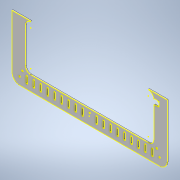
# Autodesk Inventor part: BackAcrylicPlate
Saved by Autodesk Inventor 2022 (Build 260153000, 153)
## iProperties
Created: 2021-04-22
Part Number: BackAcrylicPlate
Material: Generic
Document SubType Name: Modeling
Designer: Viktor
Density: 1 g/cm^3
Appearance: Default
Author: Viktor
Autodesk Inventor part; units mm, degrees
ref_plane "YZ Plane" through (0, 0, 0) normal (1, 0, 0) x (0, 1, 0)
ref_plane "XZ Plane" through (0, 0, 0) normal (0, 1, 0) x (-1, 0, 0)
ref_plane "XY Plane" through (0, 0, 0) normal (0, 0, 1) x (1, 0, 0)
sketch "Sketch1" plane through (0, 0, 0) normal (0, 0, 1) x (1, 0, 0)
  line L0 (-222.5, -24) -> (222.5, -24)
  line L1 (222.5, -24) -> (222.5, 24)
  line L2 (222.5, 24) -> (-222.5, 24)
  line L3 (-222.5, 24) -> (-222.5, -24)
  line L4 (-222.5, -24) -> (222.5, 24) construction
  line L5 (222.5, -24) -> (-222.5, 24) construction
  point P0 (0, 0)
  dimension "d0" = 445
  dimension "d1" = 48
  constraints: 12 end point, 2 midpoint, 2 parallel, 1 horizontal, 1 perpendicular
  measures "d0" distance of L1.end L2.end
  measures "d1" distance of L2.end L0.start
extrude "Extrusion1" add sketch "Sketch1" along normal blind 3
fillet "Fillet1" radius 22 2 edges at (-222.5, -24, 1.5) (222.5, -24, 1.5)
sketch "Sketch2" plane through (0, 0, 3) normal (0, 0, 1) x (1, 0, 0)
  line L0 (-311.5, 0) -> (311.5, 0) projected
  line L1 (0, -9) -> (0, 9) construction
  line L2 (-2, -9) -> (-2, 9)
  line L3 (2, 9) -> (2, -9)
  arc A0 (-2, -9) -> (2, -9) centre (0, -9) ccw
  arc A1 (2, 9) -> (-2, 9) centre (0, 9) ccw
  point P0 (0, 0)
  dimension "d5" = 18
  dimension "d6" = 2
  constraints: 8 end point, 4 point on circle, 4 tangent, 2 centre point, 1 midpoint, 1 parallel, 1 perpendicular
  measures "d5" distance of L3.start L3.end
  measures "d6" radius of A1
extrude "Extrusion2" cut sketch "Sketch2" against normal blind 3
pattern_linear "Rectangular Pattern1" count 10 spacing 20 along (-1, 0, 0) count 10 spacing 20 along (1, 0, 0) of "Extrusion2"
sketch "Sketch3" plane through (0, 0, 3) normal (0, 0, 1) x (1, 0, 0)
  arc A0 (-222.5, -2) -> (-200.5, -24) centre (-200.5, -2) ccw projected
  arc A1 (200.5, -24) -> (222.5, -2) centre (200.5, -2) ccw projected
  circle A2 centre (-200.5, -2) radius 2.25
  line L0 (0, 34.5113) -> (0, -39.0676) projected
  circle A3 centre (200.5, -2) radius 2.25
  point P0 (0, 0)
  dimension "d15" = 4.5
  constraints: 2 centre point, 1 coincident, 1 symmetric about line, 1 other
  measures "d15" diameter of A2
extrude "Extrusion3" cut sketch "Sketch3" against normal blind 3
fillet "Fillet2" radius 2 2 edges at (-222.5, 24, 1.5) (222.5, 24, 1.5)
sketch "Sketch7" plane through (0, 0, 3) normal (0, 0, 1) x (1, 0, 0)
  arc A0 (2, 9) -> (-2, 9) centre (0, 9) ccw projected
  line L0 (-2, -9) -> (-2, 9) projected
  arc A1 (-2, -9) -> (2, -9) centre (0, -9) ccw projected
  line L1 (2, 9) -> (2, -9) projected
  point P0 (0, 0)
extrude "Extrusion6" add sketch "Sketch7" against normal up to surface (3 mm away)
sketch "Sketch4" plane through (0, 0, 3) normal (0, 0, 1) x (1, 0, 0)
  circle A0 centre (-192.5, 16) radius 2.25
  line L0 (0, 33.6) -> (0, -33.6) projected
  line L1 (-222.5, 22) -> (-222.5, -2) projected
  line L2 (220.5, 24) -> (-220.5, 24) projected
  circle A1 centre (192.5, 16) radius 2.25
  circle A2 centre (0, 8) radius 2.25
  point P0 (0, 0)
  dimension "d19" = 4.5
  dimension "d20" = 30
  dimension "d21" = 8
  dimension "d24" = 4.5
  dimension "d25" = 16
  constraints: 3 centre point, 1 point on line, 1 symmetric about line, 1 other
  measures "d19" diameter of A0
  measures "d20" distance from line of L1 A0.centre
  measures "d21" distance from line of L2 A0.centre
  measures "d24" diameter of A2
  measures "d25" distance from line of L2 A2.centre
extrude "Extrusion4" cut sketch "Sketch4" against normal blind 3
sketch "Sketch6" plane through (0, 0, 3) normal (0, 0, 1) x (1, 0, 0)
  line L0 (0, -39.1505) -> (0, 35.0083) construction
  line L1 (-184, 40.8676) -> (184, 40.8676)
  line L2 (184, 40.8676) -> (184, 18)
  line L3 (184, 18) -> (-184, 18)
  line L4 (-184, 18) -> (-184, 40.8676)
  line L5 (-184, 40.8676) -> (184, 18) construction
  line L6 (184, 40.8676) -> (-184, 18) construction
  line L7 (220.5, 24) -> (-220.5, 24) projected
  point P0 (0, 0)
  point P1 (0, 29.4338)
  dimension "d26" = 6
  dimension "d27" = 368
  constraints: 12 end point, 2 midpoint, 2 parallel, 1 horizontal, 1 perpendicular, 1 point on line
  measures "d26" distance between parallel lines of L7 L3
  measures "d27" distance between parallel lines of L2 L4
extrude "Extrusion5" cut sketch "Sketch6" against normal through all
fillet "Fillet3" radius 1 2 edges at (-184, 18, 1.5) (184, 18, 1.5)
sketch "Sketch8" plane through (0, 0, 3) normal (0, 0, 1) x (1, 0, 0)
  line L0 (-222.5, 22) -> (-222.5, -2) projected
  line L1 (-222.5, 22) -> (-184, 22)
  line L2 (-184, 22) -> (-184, 151)
  line L3 (-184, 151) -> (-222.5, 151)
  line L4 (-222.5, 151) -> (-222.5, 22)
  line L5 (-184, 19) -> (-184, 24) projected
  line L6 (0, -64.6889) -> (0, 188.2392) projected
  line L7 (222.5, 22) -> (184, 22)
  line L8 (184, 22) -> (184, 151)
  line L9 (184, 151) -> (222.5, 151)
  line L10 (222.5, 151) -> (222.5, 22)
  line L11 (184, 19) -> (184, 24)
  line L12 (-184, 151) -> (-169, 151)
  line L13 (-169, 151) -> (-169, 149)
  line L14 (-169, 149) -> (-184, 149)
  line L15 (-184, 149) -> (-184, 151)
  line L16 (184, 151) -> (169, 151)
  line L17 (169, 151) -> (169, 149)
  line L18 (169, 149) -> (184, 149)
  point P0 (0, 0)
  point P1 (-184, 21.5)
  point P2 (184, 21.5)
  dimension "d33" = 129
  dimension "d34" = 15
  dimension "d35" = 2
  constraints: 32 end point, 10 symmetric about line, 4 parallel, 2 horizontal, 2 perpendicular, 2 point on line, 1 midpoint
  measures "d33" distance between parallel lines of L1 L3
  measures "d34" distance between parallel lines of L2 L13
  measures "d35" distance between parallel lines of L12 L14
extrude "Extrusion7" add sketch "Sketch8" against normal up to surface (3 mm away)
fillet "Fillet4" radius 15 2 edges at (-184, 149, 1.5) (184, 149, 1.5)
sketch "Sketch10" plane through (0, 0, 3) normal (0, 0, 1) x (1, 0, 0)
  line L0 (184, 136) -> (199, 136)
  line L1 (199, 136) -> (199, 121)
  line L2 (199, 121) -> (184, 121)
  line L3 (184, 121) -> (184, 136)
  line L4 (222.5, 151) -> (169, 151) projected
  point P0 (0, 0)
  dimension "d39" = 15
  dimension "d40" = 15
  dimension "d41" = 15
  constraints: 8 end point, 2 parallel, 1 horizontal, 1 perpendicular
  measures "d39" distance between parallel lines of L4 L0
  measures "d40" distance between parallel lines of L2 L0
  measures "d41" distance between parallel lines of L3 L1
extrude "Extrusion8" cut sketch "Sketch10" against normal blind 10
fillet "Fillet5" radius 2 3 edges at (184, 121, 1.5) (199, 121, 1.5) (199, 136, 1.5)
sketch "Sketch12" plane through (0, 0, 3) normal (0, 0, 1) x (1, 0, 0)
  circle A0 centre (-169, 33) radius 15
  line L0 (-184, 134) -> (-184, 19) projected
  arc A1 (186, 121) -> (184, 119) centre (186, 119) ccw projected
  line L1 (184, 119) -> (184, 19) projected
  arc A2 (183, 18) -> (184, 19) centre (183, 19) ccw projected
  line L2 (183, 18) -> (-183, 18) projected
  arc A3 (-184, 19) -> (-183, 18) centre (-183, 19) ccw projected
  line L3 (-184, 19) -> (-184, 134) projected
  arc A4 (-169, 149) -> (-184, 134) centre (-169, 134) ccw projected
  line L4 (-169, 149) -> (-169, 151) projected
  line L5 (-169, 151) -> (-222.5, 151) projected
  line L6 (-222.5, 151) -> (-222.5, -2) projected
  arc A5 (-222.5, -2) -> (-200.5, -24) centre (-200.5, -2) ccw projected
  line L7 (-200.5, -24) -> (200.5, -24) projected
  arc A6 (200.5, -24) -> (222.5, -2) centre (200.5, -2) ccw projected
  line L8 (222.5, -2) -> (222.5, 151) projected
  line L9 (222.5, 151) -> (169, 151) projected
  line L10 (169, 151) -> (169, 149) projected
  arc A7 (184, 134) -> (169, 149) centre (169, 134) ccw projected
  line L11 (184, 136) -> (197, 136) projected
  arc A8 (199, 134) -> (197, 136) centre (197, 134) ccw projected
  line L12 (199, 134) -> (199, 123) projected
  arc A9 (197, 121) -> (199, 123) centre (197, 123) ccw projected
  line L13 (197, 121) -> (186, 121) projected
  arc A10 (38, -9) -> (42, -9) centre (40, -9) ccw projected
  line L14 (38, -9) -> (38, 9) projected
  arc A11 (42, 9) -> (38, 9) centre (40, 9) ccw projected
  line L15 (42, 9) -> (42, -9) projected
  arc A12 (78, -9) -> (82, -9) centre (80, -9) ccw projected
  line L16 (78, -9) -> (78, 9) projected
  arc A13 (82, 9) -> (78, 9) centre (80, 9) ccw projected
  line L17 (82, 9) -> (82, -9) projected
  arc A14 (118, -9) -> (122, -9) centre (120, -9) ccw projected
  line L18 (118, -9) -> (118, 9) projected
  arc A15 (122, 9) -> (118, 9) centre (120, 9) ccw projected
  line L19 (122, 9) -> (122, -9) projected
  arc A16 (158, -9) -> (162, -9) centre (160, -9) ccw projected
  line L20 (158, -9) -> (158, 9) projected
  arc A17 (162, 9) -> (158, 9) centre (160, 9) ccw projected
  line L21 (162, 9) -> (162, -9) projected
  arc A18 (-22, -9) -> (-18, -9) centre (-20, -9) ccw projected
  line L22 (-22, -9) -> (-22, 9) projected
  arc A19 (-18, 9) -> (-22, 9) centre (-20, 9) ccw projected
  line L23 (-18, 9) -> (-18, -9) projected
  arc A20 (-42, -9) -> (-38, -9) centre (-40, -9) ccw projected
  line L24 (-42, -9) -> (-42, 9) projected
  arc A21 (-38, 9) -> (-42, 9) centre (-40, 9) ccw projected
  line L25 (-38, 9) -> (-38, -9) projected
  arc A22 (-62, -9) -> (-58, -9) centre (-60, -9) ccw projected
  line L26 (-62, -9) -> (-62, 9) projected
  arc A23 (-58, 9) -> (-62, 9) centre (-60, 9) ccw projected
  line L27 (-58, 9) -> (-58, -9) projected
  arc A24 (-82, -9) -> (-78, -9) centre (-80, -9) ccw projected
  line L28 (-82, -9) -> (-82, 9) projected
  arc A25 (-78, 9) -> (-82, 9) centre (-80, 9) ccw projected
  line L29 (-78, 9) -> (-78, -9) projected
  arc A26 (-102, -9) -> (-98, -9) centre (-100, -9) ccw projected
  line L30 (-102, -9) -> (-102, 9) projected
  arc A27 (-98, 9) -> (-102, 9) centre (-100, 9) ccw projected
  line L31 (-98, 9) -> (-98, -9) projected
  arc A28 (-122, -9) -> (-118, -9) centre (-120, -9) ccw projected
  line L32 (-122, -9) -> (-122, 9) projected
  arc A29 (-118, 9) -> (-122, 9) centre (-120, 9) ccw projected
  line L33 (-118, 9) -> (-118, -9) projected
  arc A30 (-142, -9) -> (-138, -9) centre (-140, -9) ccw projected
  line L34 (-142, -9) -> (-142, 9) projected
  arc A31 (-138, 9) -> (-142, 9) centre (-140, 9) ccw projected
  line L35 (-138, 9) -> (-138, -9) projected
  arc A32 (-162, -9) -> (-158, -9) centre (-160, -9) ccw projected
  line L36 (-162, -9) -> (-162, 9) projected
  arc A33 (-158, 9) -> (-162, 9) centre (-160, 9) ccw projected
  line L37 (-158, 9) -> (-158, -9) projected
  arc A34 (-182, -9) -> (-178, -9) centre (-180, -9) ccw projected
  line L38 (-182, -9) -> (-182, 9) projected
  arc A35 (-178, 9) -> (-182, 9) centre (-180, 9) ccw projected
  line L39 (-178, 9) -> (-178, -9) projected
  arc A36 (178, -9) -> (182, -9) centre (180, -9) ccw projected
  line L40 (178, -9) -> (178, 9) projected
  arc A37 (182, 9) -> (178, 9) centre (180, 9) ccw projected
  line L41 (182, 9) -> (182, -9) projected
  arc A38 (138, -9) -> (142, -9) centre (140, -9) ccw projected
  line L42 (138, -9) -> (138, 9) projected
  arc A39 (142, 9) -> (138, 9) centre (140, 9) ccw projected
  line L43 (142, 9) -> (142, -9) projected
  arc A40 (98, -9) -> (102, -9) centre (100, -9) ccw projected
  line L44 (98, -9) -> (98, 9) projected
  arc A41 (102, 9) -> (98, 9) centre (100, 9) ccw projected
  line L45 (102, 9) -> (102, -9) projected
  arc A42 (58, -9) -> (62, -9) centre (60, -9) ccw projected
  line L46 (58, -9) -> (58, 9) projected
  arc A43 (62, 9) -> (58, 9) centre (60, 9) ccw projected
  line L47 (62, 9) -> (62, -9) projected
  arc A44 (18, -9) -> (22, -9) centre (20, -9) ccw projected
  line L48 (18, -9) -> (18, 9) projected
  arc A45 (22, 9) -> (18, 9) centre (20, 9) ccw projected
  line L49 (22, 9) -> (22, -9) projected
  circle A46 centre (-200.5, -2) radius 2.25 projected
  circle A47 centre (200.5, -2) radius 2.25 projected
  circle A48 centre (0, 8) radius 2.25 projected
  circle A49 centre (-192.5, 16) radius 2.25 projected
  circle A50 centre (192.5, 16) radius 2.25 projected
  line L50 (183, 18) -> (-183, 18) projected
  line L51 (0, -64.6889) -> (0, 188.2392) projected
  circle A51 centre (169, 33) radius 15
  line L52 (184, 134) -> (184, 19)
  line L53 (-183, 18) -> (183, 18)
  arc A52 (183, 18) -> (184, 19) centre (183, 19) ccw
  line L54 (184, 19) -> (184, 134)
  arc A53 (142, 9) -> (138, 9) centre (140, 9) ccw
  arc A54 (162, 9) -> (158, 9) centre (160, 9) ccw
  arc A55 (182, 9) -> (178, 9) centre (180, 9) ccw
  line L55 (-183, 18) -> (183, 18)
  line L56 (184, 134) -> (184, 136) projected
  point P0 (0, 0)
  point P1 (184, 33)
  point P2 (169, 18)
  point P3 (-169, 18)
  point P4 (-184, 33)
  dimension "d45" = 30
  constraints: 11 symmetric about line, 8 end point, 8 point on circle, 6 centre point, 2 tangent, 5 other
  measures "d45" diameter of A0
extrude "Extrusion9" add sketch "Sketch12" against normal up to surface (3 mm away) contours A0 L2 A3 L0 | A51 L1 A2 L2
sketch "Sketch14" plane through (0, 0, 3) normal (0, 0, 1) x (1, 0, 0)
  arc A0 (186, 121) -> (184, 119) centre (186, 119) ccw projected
  line L0 (184, 119) -> (184, 33) projected
  arc A1 (169, 18) -> (184, 33) centre (169, 33) ccw projected
  line L1 (169, 18) -> (-169, 18) projected
  arc A2 (-184, 33) -> (-169, 18) centre (-169, 33) ccw projected
  line L2 (-184, 33) -> (-184, 134) projected
  arc A3 (-169, 149) -> (-184, 134) centre (-169, 134) ccw projected
  line L3 (-169, 149) -> (-169, 151) projected
  line L4 (-169, 151) -> (-222.5, 151) projected
  line L5 (-222.5, 151) -> (-222.5, -2) projected
  arc A4 (-222.5, -2) -> (-200.5, -24) centre (-200.5, -2) ccw projected
  line L6 (-200.5, -24) -> (200.5, -24) projected
  arc A5 (200.5, -24) -> (222.5, -2) centre (200.5, -2) ccw projected
  line L7 (222.5, -2) -> (222.5, 151) projected
  line L8 (222.5, 151) -> (169, 151) projected
  line L9 (169, 151) -> (169, 149) projected
  arc A6 (184, 134) -> (169, 149) centre (169, 134) ccw projected
  line L10 (184, 136) -> (197, 136) projected
  arc A7 (199, 134) -> (197, 136) centre (197, 134) ccw projected
  line L11 (199, 134) -> (199, 123) projected
  arc A8 (197, 121) -> (199, 123) centre (197, 123) ccw projected
  line L12 (197, 121) -> (186, 121) projected
  arc A9 (38, -9) -> (42, -9) centre (40, -9) ccw projected
  line L13 (38, -9) -> (38, 9) projected
  arc A10 (42, 9) -> (38, 9) centre (40, 9) ccw projected
  line L14 (42, 9) -> (42, -9) projected
  arc A11 (78, -9) -> (82, -9) centre (80, -9) ccw projected
  line L15 (78, -9) -> (78, 9) projected
  arc A12 (82, 9) -> (78, 9) centre (80, 9) ccw projected
  line L16 (82, 9) -> (82, -9) projected
  arc A13 (118, -9) -> (122, -9) centre (120, -9) ccw projected
  line L17 (118, -9) -> (118, 9) projected
  arc A14 (122, 9) -> (118, 9) centre (120, 9) ccw projected
  line L18 (122, 9) -> (122, -9) projected
  arc A15 (158, -9) -> (162, -9) centre (160, -9) ccw projected
  line L19 (158, -9) -> (158, 9) projected
  arc A16 (162, 9) -> (158, 9) centre (160, 9) ccw projected
  line L20 (162, 9) -> (162, -9) projected
  arc A17 (-22, -9) -> (-18, -9) centre (-20, -9) ccw projected
  line L21 (-22, -9) -> (-22, 9) projected
  arc A18 (-18, 9) -> (-22, 9) centre (-20, 9) ccw projected
  line L22 (-18, 9) -> (-18, -9) projected
  arc A19 (-42, -9) -> (-38, -9) centre (-40, -9) ccw projected
  line L23 (-42, -9) -> (-42, 9) projected
  arc A20 (-38, 9) -> (-42, 9) centre (-40, 9) ccw projected
  line L24 (-38, 9) -> (-38, -9) projected
  arc A21 (-62, -9) -> (-58, -9) centre (-60, -9) ccw projected
  line L25 (-62, -9) -> (-62, 9) projected
  arc A22 (-58, 9) -> (-62, 9) centre (-60, 9) ccw projected
  line L26 (-58, 9) -> (-58, -9) projected
  arc A23 (-82, -9) -> (-78, -9) centre (-80, -9) ccw projected
  line L27 (-82, -9) -> (-82, 9) projected
  arc A24 (-78, 9) -> (-82, 9) centre (-80, 9) ccw projected
  line L28 (-78, 9) -> (-78, -9) projected
  arc A25 (-102, -9) -> (-98, -9) centre (-100, -9) ccw projected
  line L29 (-102, -9) -> (-102, 9) projected
  arc A26 (-98, 9) -> (-102, 9) centre (-100, 9) ccw projected
  line L30 (-98, 9) -> (-98, -9) projected
  arc A27 (-122, -9) -> (-118, -9) centre (-120, -9) ccw projected
  line L31 (-122, -9) -> (-122, 9) projected
  arc A28 (-118, 9) -> (-122, 9) centre (-120, 9) ccw projected
  line L32 (-118, 9) -> (-118, -9) projected
  arc A29 (-142, -9) -> (-138, -9) centre (-140, -9) ccw projected
  line L33 (-142, -9) -> (-142, 9) projected
  arc A30 (-138, 9) -> (-142, 9) centre (-140, 9) ccw projected
  line L34 (-138, 9) -> (-138, -9) projected
  arc A31 (-162, -9) -> (-158, -9) centre (-160, -9) ccw projected
  line L35 (-162, -9) -> (-162, 9) projected
  arc A32 (-158, 9) -> (-162, 9) centre (-160, 9) ccw projected
  line L36 (-158, 9) -> (-158, -9) projected
  arc A33 (-182, -9) -> (-178, -9) centre (-180, -9) ccw projected
  line L37 (-182, -9) -> (-182, 9) projected
  arc A34 (-178, 9) -> (-182, 9) centre (-180, 9) ccw projected
  line L38 (-178, 9) -> (-178, -9) projected
  arc A35 (178, -9) -> (182, -9) centre (180, -9) ccw projected
  line L39 (178, -9) -> (178, 9) projected
  arc A36 (182, 9) -> (178, 9) centre (180, 9) ccw projected
  line L40 (182, 9) -> (182, -9) projected
  arc A37 (138, -9) -> (142, -9) centre (140, -9) ccw projected
  line L41 (138, -9) -> (138, 9) projected
  arc A38 (142, 9) -> (138, 9) centre (140, 9) ccw projected
  line L42 (142, 9) -> (142, -9) projected
  arc A39 (98, -9) -> (102, -9) centre (100, -9) ccw projected
  line L43 (98, -9) -> (98, 9) projected
  arc A40 (102, 9) -> (98, 9) centre (100, 9) ccw projected
  line L44 (102, 9) -> (102, -9) projected
  arc A41 (58, -9) -> (62, -9) centre (60, -9) ccw projected
  line L45 (58, -9) -> (58, 9) projected
  arc A42 (62, 9) -> (58, 9) centre (60, 9) ccw projected
  line L46 (62, 9) -> (62, -9) projected
  arc A43 (18, -9) -> (22, -9) centre (20, -9) ccw projected
  line L47 (18, -9) -> (18, 9) projected
  arc A44 (22, 9) -> (18, 9) centre (20, 9) ccw projected
  line L48 (22, 9) -> (22, -9) projected
  circle A45 centre (-200.5, -2) radius 2.25 projected
  circle A46 centre (200.5, -2) radius 2.25 projected
  circle A47 centre (0, 8) radius 2.25 projected
  circle A48 centre (-192.5, 16) radius 2.25 projected
  circle A49 centre (192.5, 16) radius 2.25 projected
  line L49 (184, 134) -> (184, 136) projected
  point P0 (0, 0)
equation "\"d24\" = d19"
body "Solid1"
